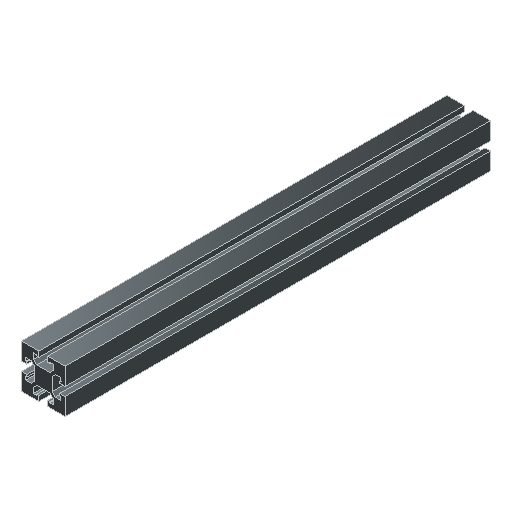
# Autodesk Inventor part: 39
Saved by Autodesk Inventor 2025.2 (Build 292293000, 293)
## iProperties
Created: 2024-02-07
Part Number: 39
Material: 철, 회색
Document SubType Name: Modeling
Designer: ps737
Density: 7.15 g/cm^3
Appearance: 철 회색
Mass: 2650.14 g
Surface Area: 1334.66 cm^2
Volume: 370.649 cm^3
Author: ps737
Autodesk Inventor part; units mm, degrees
ref_plane "YZ Plane" through (0, 0, 0) normal (1, 0, 0) x (0, 1, 0)
ref_plane "XZ Plane" through (0, 0, 0) normal (0, 1, 0) x (-1, 0, 0)
ref_plane "XY Plane" through (0, 0, 0) normal (0, 0, 1) x (1, 0, 0)
sketch "스케치1" plane through (0, 0, 0) normal (0, 0, 1) x (1, 0, 0)
  line L0 (40, 40) -> (25, 40)
  line L1 (15, 40) -> (0, 40)
  line L2 (16, 40) -> (16, 35)
  line L3 (16, 35) -> (14, 35)
  line L4 (14, 35) -> (14, 36)
  line L5 (14, 36) -> (11, 36)
  line L6 (11, 36) -> (11, 31)
  line L7 (11, 31) -> (14, 28)
  line L8 (11, 31) -> (20.81, 31) construction
  line L9 (14, 28) -> (20, 28)
  line L10 (24, 40) -> (24, 35)
  line L11 (24, 35) -> (26, 35)
  line L12 (26, 35) -> (26, 36)
  line L13 (26, 36) -> (29, 36)
  line L14 (29, 36) -> (29, 31)
  line L15 (29, 31) -> (26, 28)
  line L16 (29, 31) -> (19.19, 31) construction
  line L17 (26, 28) -> (20, 28)
  line L18 (-0.0744, 15.9256) -> (4.9256, 15.9256)
  line L19 (-0.0744, 23.9256) -> (4.9256, 23.9256)
  line L20 (4.9256, 23.9256) -> (4.9256, 25.9256)
  line L21 (11.9256, 25.9256) -> (11.9256, 19.9256)
  line L22 (8.9256, 28.9256) -> (8.9256, 19.1155) construction
  line L23 (8.9256, 28.9256) -> (11.9256, 25.9256)
  line L24 (3.9256, 28.9256) -> (8.9256, 28.9256)
  line L25 (3.9256, 25.9256) -> (3.9256, 28.9256)
  line L26 (4.9256, 25.9256) -> (3.9256, 25.9256)
  line L27 (4.9256, 15.9256) -> (4.9256, 13.9256)
  line L28 (11.9256, 13.9256) -> (11.9256, 19.9256)
  line L29 (4.9256, 13.9256) -> (3.9256, 13.9256)
  line L30 (8.9256, 10.9256) -> (11.9256, 13.9256)
  line L31 (8.9256, 10.9256) -> (8.9256, 20.7356) construction
  line L32 (3.9256, 13.9256) -> (3.9256, 10.9256)
  line L33 (3.9256, 10.9256) -> (8.9256, 10.9256)
  line L34 (24, -0.1488) -> (24, 4.8512)
  line L35 (16, -0.1488) -> (16, 4.8512)
  line L36 (16, 4.8512) -> (14, 4.8512)
  line L37 (14, 11.8512) -> (20, 11.8512)
  line L38 (11, 8.8512) -> (20.81, 8.8512) construction
  line L39 (11, 8.8512) -> (14, 11.8512)
  line L40 (11, 3.8512) -> (11, 8.8512)
  line L41 (14, 3.8512) -> (11, 3.8512)
  line L42 (14, 4.8512) -> (14, 3.8512)
  line L43 (24, 4.8512) -> (26, 4.8512)
  line L44 (26, 11.8512) -> (20, 11.8512)
  line L45 (26, 4.8512) -> (26, 3.8512)
  line L46 (29, 8.8512) -> (26, 11.8512)
  line L47 (29, 8.8512) -> (19.19, 8.8512) construction
  line L48 (26, 3.8512) -> (29, 3.8512)
  line L49 (29, 3.8512) -> (29, 8.8512)
  line L50 (40.0744, 23.9256) -> (35.0744, 23.9256)
  line L51 (40.0744, 15.9256) -> (35.0744, 15.9256)
  line L52 (35.0744, 15.9256) -> (35.0744, 13.9256)
  line L53 (28.0744, 13.9256) -> (28.0744, 19.9256)
  line L54 (31.0744, 10.9256) -> (31.0744, 20.7356) construction
  line L55 (31.0744, 10.9256) -> (28.0744, 13.9256)
  line L56 (36.0744, 10.9256) -> (31.0744, 10.9256)
  line L57 (36.0744, 13.9256) -> (36.0744, 10.9256)
  line L58 (35.0744, 13.9256) -> (36.0744, 13.9256)
  line L59 (35.0744, 23.9256) -> (35.0744, 25.9256)
  line L60 (28.0744, 25.9256) -> (28.0744, 19.9256)
  line L61 (35.0744, 25.9256) -> (36.0744, 25.9256)
  line L62 (31.0744, 28.9256) -> (28.0744, 25.9256)
  line L63 (31.0744, 28.9256) -> (31.0744, 19.1155) construction
  line L64 (36.0744, 25.9256) -> (36.0744, 28.9256)
  line L65 (36.0744, 28.9256) -> (31.0744, 28.9256)
  line L66 (11, 20) -> (11.9256, 20)
  line L67 (28.0744, 20) -> (29, 20)
  line L68 (20, 3.8512) -> (20, 4.8512)
  line L69 (20, 35) -> (20, 36)
  line L70 (15, 40) -> (16, 40)
  line L71 (24, 40) -> (25, 40)
  line L72 (0, 40) -> (0, 23.9256)
  line L73 (0, 15.9256) -> (0, 0)
  line L74 (40, 0) -> (40, 15.9256)
  line L75 (40, 23.9256) -> (40, 40)
  line L76 (0, 0) -> (16, 0)
  line L77 (24, 0) -> (40, 0)
  point P0 (25, 38)
  point P1 (20, 19.9256)
  point P2 (15, 35)
  point P3 (25, 35)
  point P4 (4.9256, 24.9256)
  point P5 (4.9256, 14.9256)
  point P6 (15, 4.8512)
  point P7 (25, 4.8512)
  point P8 (35.0744, 14.9256)
  point P9 (35.0744, 24.9256)
  dimension "d0" = 40
  dimension "d1" = 40
  dimension "d14" = 2
  dimension "d15" = 5
  dimension "d16" = 1
  dimension "d17" = 3
  dimension "d18" = 5
  dimension "d19" = 45
  dimension "d21" = 7
  dimension "d24" = 360
  constraints: 156 end point, 14 point on line, 9 perpendicular, 8 parallel, 4 vertical, 3 horizontal, 1 midpoint, 141 other
  measures "d0" distance of L1.end L0.start
  measures "d1" distance of L0.start L74.start
  measures "d14" distance of L2.end L3.end
  measures "d15" distance from line of point (15, 35) L1
  measures "d16" distance of L3.end L4.end
  measures "d17" distance of L4.end L5.end
  measures "d18" distance of L5.end L6.end
  measures "d19" angle of L7 L8
  measures "d21" distance between parallel lines of L9 L3
extrude "돌출1" add sketch "스케치1" along normal mid plane 390
